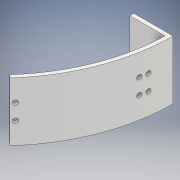
# Autodesk Inventor part: CW005
Saved by Autodesk Inventor 2017 SP1 (Build 210196100, 196)
## iProperties
Created: 2017-05-24
Part Number: CW005
Material: ABS Plastic
Document SubType Name: Modeling
Designer: zallen
Density: 1.06 g/cm^3
Appearance: CR White
Author: zallen
Autodesk Inventor part; units mm, degrees
ref_plane "YZ Plane" through (0, 0, 0) normal (1, 0, 0) x (0, 1, 0)
sketch "Sketch1" plane through (0, 0, 0) normal (0, 0, 1) x (1, 0, 0)
  line L0 (0, 0) -> (-50, 0)
  line L1 (-50, 0) -> (-50, 5)
  line L2 (-50, 5) -> (0, 5)
  line L3 (0, 5) -> (0, 0)
  dimension "d0" = 50
  dimension "d1" = 5
  constraints: 8 end point, 2 parallel, 1 horizontal, 1 perpendicular
  measures "d0" distance of L1.end L2.end
  measures "d1" distance of L0.end L1.end
extrude "Extrusion1" add sketch "Sketch1" along normal blind 75
sketch "Sketch2" plane through (0, 0, 75) normal (0, 0, 1) x (1, 0, 0)
  circle A0 centre (-225, 5) radius 225 construction
  circle A1 centre (-225, 5) radius 220 construction
  line L0 (0, 0) -> (0, 5) projected
  line L1 (0, 5) -> (-5, 5)
  arc A2 (-57.7435, -145.5) -> (0, 5) centre (-225, 5) ccw
  line L2 (-57.7435, -145.5) -> (-61.4603, -142.1556)
  arc A3 (-61.4603, -142.1556) -> (-5, 5) centre (-225, 5) ccw
  dimension "d4" = 450
  dimension "d5" = 5
  dimension "d6" = 5
  dimension "d7" = 150.5
  constraints: 8 point on circle, 4 centre point, 4 end point, 2 concentric, 1 horizontal alignment, 1 perpendicular
  measures "d4" diameter of A0
  measures "d5" radial gap between concentric circles of A0 A1
  measures "d6" distance of L2.start L2.end
  measures "d7" vertical distance of L2.start L0.end
extrude "Extrusion2" add sketch "Sketch2" against normal blind 75
sketch "Sketch3" plane through (-50, 5, 0) normal (0, 1, 0) x (1, 0, 0)
  line L0 (45, -10) -> (5, -10)
  line L1 (5, -10) -> (5, -12)
  line L2 (5, -12) -> (45, -12)
  line L3 (45, -12) -> (45, -10)
  line L4 (0, 0) -> (0, -75) projected
  line L5 (0, 0) -> (50, 0) projected
  line L6 (5, -17) -> (45, -17)
  line L7 (45, -17) -> (45, -15)
  line L8 (45, -15) -> (5, -15)
  line L9 (5, -15) -> (5, -17)
  line L10 (5, -22) -> (45, -22)
  line L11 (45, -22) -> (45, -20)
  line L12 (45, -20) -> (5, -20)
  line L13 (5, -20) -> (5, -22)
  dimension "d10" = 40
  dimension "d11" = 2
  dimension "d12" = 5
  dimension "d13" = 10
  dimension "d16" = 5
  constraints: 24 end point, 2 parallel, 1 horizontal, 1 perpendicular, 1 vertical, 16 other
  measures "d10" distance of L2.end L1.end
  measures "d11" distance of L0.end L1.end
  measures "d12" distance from line of L4 L0.end
  measures "d13" distance from line of L5 L0.end
  measures "d16" distance of L1.end L6.start
extrude "Extrusion3" cut sketch "Sketch3" against normal blind 5
ref_plane "Work Plane1" through (0, 5, 0) normal (1, 0, 0) x (0, 1, 0)
sketch "Sketch4" plane through (0, 5, 0) normal (1, 0, 0) x (0, 1, 0)
  circle A0 centre (-29.5, 47.5) radius 3
  circle A1 centre (-29.5, 27.5) radius 3
  line L0 (-5, 0) -> (-5, 75) projected
  line L1 (-150.5, 0) -> (-5, 0) projected
  circle A2 centre (-39.5, 47.5) radius 3
  circle A3 centre (-39.5, 27.5) radius 3
  line L2 (0, 0) -> (0, 75) projected
  dimension "d23" = 6
  dimension "d24" = 6
  dimension "d26" = 27.5
  dimension "d27" = 20
  dimension "d30" = 6
  dimension "d31" = 6
  dimension "d32" = 10
  dimension "d33" = 29.5
  constraints: 4 centre point, 2 horizontal alignment, 2 vertical alignment
  measures "d23" diameter of A0
  measures "d24" diameter of A1
  measures "d26" distance from line of L1 A1.centre
  measures "d27" distance of A1.centre A0.centre
  measures "d30" diameter of A2
  measures "d31" diameter of A3
  measures "d32" distance of A1.centre A3.centre
  measures "d33" distance from line of A1.centre L2
extrude "Extrusion4" cut sketch "Sketch4" along normal through all both and the other way through all
ref_plane "Work Plane2" through (-57.7435, -145.5, 75) normal (0.7434, -0.6689, 0) x (0.6689, 0.7434, 0)
sketch "Sketch5" plane through (-57.7435, -145.5, 75) normal (0.7434, -0.6689, 0) x (0.6689, 0.7434, 0)
  circle A0 centre (5, -27.5) radius 3
  circle A1 centre (5, -47.5) radius 3
  line L0 (0, 0) -> (0, -75) projected
  line L1 (0, -75) -> (146.746, -75) projected
  point P0 (146.7832, -75)
  dimension "d34" = 6
  dimension "d35" = 6
  dimension "d36" = 5
  dimension "d37" = 27.5
  dimension "d38" = 20
  constraints: 2 centre point, 1 vertical alignment
  measures "d34" diameter of A0
  measures "d35" diameter of A1
  measures "d36" distance from line of L0 A1.centre
  measures "d37" distance from line of L1 A1.centre
  measures "d38" distance of A0.centre A1.centre
extrude "Extrusion5" cut sketch "Sketch5" along normal through all both and the other way through all
sketch "Sketch6" plane through (-50, 0, 0) normal (-1, 0, 0) x (0, 0, 1)
  circle A0 centre (47.5, 2.5) radius 1
  circle A1 centre (27.5, 2.5) radius 1
  line L0 (0, 0) -> (0, 5) projected
  line L1 (0, 5) -> (75, 5) projected
  dimension "d41" = 2
  dimension "d42" = 2
  dimension "d43" = 27.5
  dimension "d44" = 20
  dimension "d45" = 2.5
  constraints: 2 centre point, 1 horizontal alignment
  measures "d41" diameter of A0
  measures "d42" diameter of A1
  measures "d43" distance from line of L0 A1.centre
  measures "d44" distance of A0.centre A1.centre
  measures "d45" distance from line of L1 A1.centre
extrude "Extrusion6" cut sketch "Sketch6" against normal blind 10
thread "Thread1" size "M2x0.4" class "6H" standard "ANSI Metric M Profile" full length
thread "Thread2" size "M2x0.4" class "6H" standard "ANSI Metric M Profile" full length
sketch "Sketch7" plane through (0, 0, 75) normal (0, 0, 1) x (1, 0, 0)
  circle A0 centre (-225, 5) radius 225
  circle A1 centre (-225, 5) radius 230
  point P0 (0, 0)
  point P1 (0, 5)
  dimension "d52" = 450
  dimension "d53" = 5
  constraints: 2 horizontal alignment, 1 centre point, 2 other
extrude "Extrusion7" cut sketch "Sketch7" against normal through all
body "Solid1"
